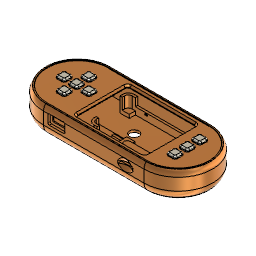
Plus_Reference (Autodesk Fusion 360 design; units mm, degrees)
Autodesk Fusion 360 part; units mm, degrees
note: some values were not read from the file. Chosen so that the rebuilt part matches the saved one: a side. Set by a fixed rule: which sketch regions a step uses.
(part 1 of 2)
sketch "Sketch1" plane through (0, 0, 0) normal (0, 0, 1) x (1, 0, 0)
  line L0 (42.95, 29.25) -> (-42.95, 29.25)
  arc A0 (-42.95, 29.25) -> (-42.95, -29.25) centre (-42.95, 0) ccw
  line L1 (-42.95, -29.25) -> (42.95, -29.25)
  arc A1 (42.95, -29.25) -> (42.95, 29.25) centre (42.95, 0) ccw
  line L2 (-42.95, 26.25) -> (42.95, 26.25)
  arc A2 (-42.95, 26.25) -> (-42.95, -26.25) centre (-42.95, 0) ccw
  line L3 (42.95, -26.25) -> (-42.95, -26.25)
  arc A3 (42.95, -26.25) -> (42.95, 26.25) centre (42.95, 0) ccw
extrude "Extrude1" add sketch "Sketch1" along normal blind 2.5 contours L2 A2 L3 A3 makes body 1
extrude "Extrude2" add sketch "Sketch1" along normal blind 22.25 bodies 1
sketch "Sketch2" plane through (0, 0, 2.5) normal (0, 0, 1) x (-1, 0, 0)
  arc A0 (42.95, -26.25) -> (42.95, 26.25) centre (42.95, 0) ccw
  line L0 (42.95, 26.25) -> (-42.95, 26.25)
  arc A1 (-42.95, 26.25) -> (-42.95, -26.25) centre (-42.95, 0) ccw
  line L1 (-42.95, -26.25) -> (42.95, -26.25)
  circle A2 centre (2.5662, -7.8588) radius 4
  arc A3 (-40.2014, 10.4179) -> (-45.3243, 5.1694) centre (-40.0743, 5.1694) ccw
  line L2 (-40.1743, 8.4179) -> (18.6467, 8.4179)
  arc A4 (-40.1743, 8.4179) -> (-43.3243, 5.1694) centre (-40.0743, 5.1694) ccw
  arc A5 (21.8967, 5.1679) -> (18.6467, 8.4179) centre (18.6467, 5.1679) ccw
  line L3 (15.8967, -22.2291) -> (15.8967, 10.4179)
  line L4 (-37.3243, -22.2291) -> (-37.3243, -24.2291)
  line L5 (-37.3243, -16.9791) -> (-37.3243, -22.2291)
  line L6 (15.8967, -22.2291) -> (15.8967, -24.2291)
  line L7 (-43.3243, -16.9791) -> (-37.3243, -16.9791)
  line L8 (21.8967, -18.9791) -> (21.8967, -15.0806)
  arc A6 (23.8967, 5.1679) -> (18.6467, 10.4179) centre (18.6467, 5.1679) ccw
  line L9 (-37.3243, -22.2291) -> (-37.3243, 10.4179)
  line L10 (-43.3243, -16.9791) -> (21.8967, -16.9791) construction
  line L11 (23.8967, -3.0806) -> (23.8967, 5.1679)
  line L12 (-40.0743, -22.2291) -> (-37.3243, -22.2291)
  line L13 (21.8967, 3.1694) -> (23.8967, 3.1694)
  line L14 (-45.3243, 3.1694) -> (-45.3243, 5.1694)
  line L15 (15.8967, -24.2291) -> (18.6467, -24.2291)
  arc A7 (18.6467, -24.2291) -> (23.8967, -18.9791) centre (18.6467, -18.9791) ccw
  line L16 (23.8967, -18.9791) -> (23.8967, -15.0806)
  line L17 (15.8967, -22.2291) -> (18.6467, -22.2291)
  line L18 (-43.3243, 3.1694) -> (21.8967, 3.1694)
  arc A8 (-45.3243, -18.9791) -> (-40.0743, -24.2291) centre (-40.0743, -18.9791) ccw
  line L19 (-45.3243, -16.9791) -> (-45.3243, -18.9791)
  line L20 (-43.3243, 3.1694) -> (-43.3243, 5.1694)
  line L21 (-40.0743, -24.2291) -> (-37.3243, -24.2291)
  line L22 (-45.3243, 3.1694) -> (-43.3243, 3.1694)
  line L23 (21.8967, -16.9791) -> (23.8967, -16.9791)
  line L24 (-40.2014, 10.4179) -> (18.6467, 10.4179)
  line L25 (15.8967, -16.9791) -> (15.8967, -22.2291)
  line L26 (15.8967, -22.2291) -> (-37.3243, -22.2291)
  line L27 (21.8967, -3.0806) -> (21.8967, -15.0806)
  arc A9 (18.6467, -22.2291) -> (21.8967, -18.9791) centre (18.6467, -18.9791) ccw
  line L28 (15.8967, -24.2291) -> (-37.3243, -24.2291)
  arc A10 (-43.3243, -18.9791) -> (-40.0743, -22.2291) centre (-40.0743, -18.9791) ccw
  line L29 (-45.3243, -16.9791) -> (-43.3243, -16.9791)
  line L30 (21.8967, -3.0806) -> (21.8967, 5.1679)
  line L31 (23.8967, -3.0806) -> (23.8967, -15.0806)
  line L32 (-43.3243, -16.9791) -> (-43.3243, -18.9791)
  line L33 (21.8967, -16.9791) -> (15.8967, -16.9791)
  arc A11 (42.95, -23.25) -> (42.95, 23.25) centre (42.95, 0) ccw
  arc A12 (42.95, -21.25) -> (42.95, 21.25) centre (42.95, 0) ccw
  arc A13 (-42.95, 23.25) -> (-42.95, -23.25) centre (-42.95, 0) ccw
  arc A14 (-42.95, 21.25) -> (-42.95, -21.25) centre (-42.95, 0) ccw
  line L34 (42.95, -23.25) -> (42.95, -21.25)
  line L35 (42.95, 21.25) -> (42.95, 23.25)
  line L36 (-42.95, 21.25) -> (-42.95, 23.25)
  line L37 (-42.95, 0) -> (-63.0851, -11.625)
  line L38 (-42.95, 0) -> (-19.7, 0) construction
  line L39 (-42.95, 0) -> (-63.0851, 11.625)
  line L40 (-42.95, 0) -> (-19.7, 0) construction
  line L41 (42.95, 0) -> (63.0851, -11.625)
  line L42 (42.95, 0) -> (66.2, 0) construction
  line L43 (42.95, 0) -> (63.0851, 11.625)
  line L44 (42.95, 0) -> (66.2, 0) construction
  line L45 (-16.3504, 12.3135) -> (-13.7656, 12.3135)
  arc A15 (-13.7656, 12.3135) -> (-13.7656, 17.551) centre (-14.2529, 14.9323) ccw
  line L46 (-13.7656, 17.551) -> (-16.0557, 17.6179)
  line L47 (-16.0557, 17.6179) -> (-16.4158, 18.1418)
  line L48 (-39.6855, 12.3135) -> (-37.1008, 12.3135)
  arc A16 (-39.6855, 17.551) -> (-39.6855, 12.3135) centre (-39.1982, 14.9323) ccw
  line L49 (-37.3955, 17.6179) -> (-39.6855, 17.551)
  line L50 (-37.0353, 18.1418) -> (-37.3955, 17.6179)
  line L51 (-16.3504, 12.3135) -> (-16.3504, 10.4179)
  line L52 (-37.1008, 12.3135) -> (-37.1008, 10.4179)
  line L53 (-16.4158, 18.1418) -> (-16.4158, 26.25)
  line L54 (-37.0353, 18.1418) -> (-37.0353, 26.25)
  line L55 (-9.4158, 26.25) -> (-9.4158, 10.4179)
  line L56 (-44.0353, 23.2247) -> (-44.0353, 26.2276)
  line L57 (-44.0353, 21.2223) -> (-44.0353, 8.6151)
  point P0 (-42.95, 0)
  point P1 (-45.1535, 0.568)
  dimension "d5" = 2
  dimension "d6" = 6
  dimension "d7" = 6
  dimension "d8" = 8
  dimension "d11" = -3
  dimension "d12" = -5
  dimension "d13" = -3
  dimension "d14" = -5
  dimension "d15" = 150
  dimension "d16" = 150
  dimension "d17" = 30
  dimension "d18" = 30
  constraint parallel L8 L27
  constraint perpendicular L20 L22
  constraint perpendicular L29 L32
  constraint coincident L13.start L30
  constraint perpendicular L18 L30
  constraint coincident L10.end L8
  constraint perpendicular L8 L10
  constraint perpendicular L7 L32
  constraint coincident L4.start L26
  constraint coincident L4.start L12
  constraint horizontal L23
  constraint coincident L23.end L16
  constraint perpendicular L16 L23
  constraint coincident L13.end L11
  constraint perpendicular L11 L13
  constraint perpendicular L6 L28
  constraint coincident L3.end L24
  constraint perpendicular L3 L24
  constraint perpendicular L4 L28
  constraint coincident L9.end L24
  constraint perpendicular L9 L24
  constraint perpendicular L1 L34
  constraint vertical L35
  constraint vertical L36
  constraint horizontal L38
  constraint coincident P0 A1.centre
  constraint coincident A13 L37.end
  constraint horizontal L40
  constraint coincident A13 L39.end
  constraint horizontal L42
  constraint coincident A0.centre A11.centre
  constraint coincident A11 L41.end
  constraint horizontal L44
  constraint coincident A11 L43.end
  constraint vertical L51
  constraint coincident L24 L51.end
  constraint perpendicular L24 L51
  constraint vertical L52
  constraint coincident L24 L52.end
  constraint vertical L53
  constraint coincident L0 L53.end
  constraint vertical L54
  constraint coincident L0 L54.end
  constraint vertical L55
  constraint coincident L24 L55.end
  constraint coincident A1 L56.end
  constraint coincident A13 L56.start
  constraint vertical L57
  constraint coincident A14 L57.start
  constraint coincident A3 L57.end
  measures "d6" distance of L10.end L25.start
  measures "d7" distance of L7.start L5.start
  measures "d8" diameter of A2
  measures "d15" angle of L37 L38
  measures "d16" angle of L39 L40
  measures "d17" angle of L41 L42
  measures "d18" angle of L43 L44
extrude "Extrude3" add sketch "Sketch2" along normal blind 3 contours L2 L3 L9 L18 | L2 A5 L3 L18 L30 | L2 A4 L9 L18 L20 | L3 L8 L17 L25 A9 L33 | L5 L7 L9 L12 A10 L32 bodies 1
extrude "Extrude4" add sketch "Sketch2" along normal blind 12.75 contours A13 A14 L36 L39 | A8 A13 A14 L37 | L4 L12 A8 L19 L21 A10 L29 L32 | L6 L8 L15 A7 L16 L17 L23 A9 | A11 A12 L34 L41 | A11 A12 L35 L43 bodies 1
extrude "Extrude5" add sketch "Sketch2" along normal blind 7.5 contours L2 L3 L9 L24 | L2 A5 L3 A6 L11 L13 L24 L30 | A3 L2 A4 L9 L14 L20 L22 L24 bodies 1
extrude "Extrude6" add sketch "Sketch2" along normal blind 6 contours L4 L6 L26 L28 bodies 1
extrude "Extrude12" add sketch "Sketch2" along normal blind 7.5 contours L0 L24 L45 A15 L46 L47 L48 A16 L49 L50 L51 L52 L53 L54 bodies 1
extrude "Extrude13" add sketch "Sketch2" along normal blind 12.75 contours L0 L24 L45 A15 L46 L47 L51 L53 L55 | L0 A1 A3 L24 A13 A14 L36 L48 A16 L49 L50 L52 L54 L56 L57 bodies 1
extrude "Extrude16" cut sketch "Sketch2" against normal up to surface (2.5 mm away) contours A2 bodies 1
sketch "Sketch3" plane through (0, -8.4179, 0) normal (0, 1, 0) x (-1, 0, 0)
  line L0 (-40.1743, 5.5) -> (18.6467, 5.5)
  line L1 (18.6467, 5.5) -> (18.6467, 10)
  line L2 (18.6467, 10) -> (-40.1743, 10)
  line L3 (-40.1743, 10) -> (-40.1743, 5.5)
  line L4 (-27.4484, 8.7376) -> (-27.4474, 8.166)
  line L5 (-27.4484, 9.136) -> (-27.4484, 8.7376)
  arc A0 (-34.511, 6.0757) -> (-34.073, 5.8861) centre (-34.0732, 6.4861) ccw
  arc A1 (-27.6097, 7.7546) -> (-27.4474, 8.166) centre (-28.0474, 8.1649) ccw
  arc A2 (-36.2473, 8.1651) -> (-36.085, 7.7547) centre (-35.6473, 8.1651) ccw
  line L6 (3.4969, 6.2998) -> (3.4969, 10.4998)
  line L7 (-25.0533, 6.7) -> (-27.0533, 6.7)
  line L8 (-31.7563, 5.887) -> (-34.073, 5.8861)
  line L9 (15.9969, 10.4998) -> (15.9969, 6.2998)
  line L10 (-27.0533, 6.7) -> (-27.0533, 7.7)
  line L11 (-34.511, 6.0757) -> (-36.085, 7.7547)
  line L12 (-36.2473, 9.136) -> (-27.4484, 9.136)
  line L13 (15.9969, 6.2998) -> (3.4969, 6.2998)
  line L14 (-0.0033, 6.7) -> (-0.0033, 7.7)
  line L15 (1.9967, 7.7) -> (1.9967, 6.7)
  line L16 (-36.2473, 8.1651) -> (-36.2473, 9.136)
  line L17 (1.9967, 6.7) -> (-0.0033, 6.7)
  line L18 (-15.0031, 5.7998) -> (-23.5031, 5.7998)
  line L19 (-27.0533, 5.5) -> (-27.0533, 6.7) construction
  line L20 (-29.6216, 5.8861) -> (-31.7563, 5.887)
  line L21 (-15.0031, 10.0008) -> (-15.0031, 5.7998)
  line L22 (-25.0533, 7.7) -> (-25.0533, 6.7)
  line L23 (-23.5031, 10.0008) -> (-15.0031, 10.0008)
  line L24 (-27.0533, 7.7) -> (-25.0533, 7.7)
  arc A3 (-29.6216, 5.8861) -> (-29.1836, 6.0757) centre (-29.6213, 6.4861) ccw
  line L25 (-0.0033, 7.7) -> (1.9967, 7.7)
  line L26 (-27.6097, 7.7546) -> (-29.1836, 6.0757)
  line L27 (-23.5031, 5.7998) -> (-23.5031, 10.0008)
  line L28 (3.4969, 10.4998) -> (15.9969, 10.4998)
  line L29 (-40.1743, 5.5) -> (-36.7473, 5.5)
  dimension "d25" = 3.427
  dimension "d26" = 1.2
  dimension "d27" = 2
  dimension "d28" = 1
  dimension "d29" = 2
  dimension "d30" = 1
  constraint vertical L19
  constraint horizontal L17
  constraint vertical L14
  constraint horizontal L25
  constraint vertical L15
  constraint horizontal L7
  constraint vertical L10
  constraint horizontal L24
  constraint vertical L22
  measures "d25" distance of L29.end L0.start
  measures "d26" distance of L19.start L7.end
  measures "d27" distance of L14.start L15.end
  measures "d28" distance of L15.start L15.end
  measures "d29" distance of L7.end L7.start
  measures "d30" distance of L7.start L22.start
extrude "Extrude7" cut sketch "Sketch3" against normal up to surface (2 mm away) contours L2 L18 L21 L23 L27 | L2 L6 L9 L13 | L2 L6 L9 L28 | L4 L5 A0 A1 A2 L8 L11 L12 L16 L20 A3 L26 bodies 1
extrude "Extrude8" add sketch "Sketch3" along normal blind 0.5 contours L7 L10 L22 L24 | L14 L15 L17 L25 bodies 1
sketch "Sketch4" plane through (0, 22.2291, 0) normal (0, -1, 0) x (1, 0, 0)
  line L0 (-18.6467, 5.5) -> (-15.8967, 5.5)
  line L1 (-15.8967, 5.5) -> (-15.8967, 2.5)
  line L2 (-15.8967, 2.5) -> (37.3243, 2.5)
  line L3 (37.3243, 2.5) -> (37.3243, 5.5)
  line L4 (37.3243, 5.5) -> (40.0743, 5.5)
  line L5 (40.0743, 5.5) -> (40.0743, 15.25)
  line L6 (40.0743, 15.25) -> (37.3243, 15.25)
  line L7 (37.3243, 15.25) -> (37.3243, 8.5)
  line L8 (37.3243, 8.5) -> (-15.8967, 8.5)
  line L9 (-15.8967, 8.5) -> (-15.8967, 15.25)
  line L10 (-15.8967, 15.25) -> (-18.6467, 15.25)
  line L11 (-18.6467, 15.25) -> (-18.6467, 5.5)
  line L12 (29.4019, 7.7) -> (27.4019, 7.7)
  line L13 (27.4019, 6.7) -> (29.4019, 6.7)
  line L14 (27.4019, 7.7) -> (27.4019, 6.7)
  line L15 (29.4019, 6.7) -> (29.4019, 7.7)
  line L16 (-5.5981, 7.7) -> (-7.5981, 7.7)
  line L17 (-7.5981, 6.7) -> (-5.5981, 6.7)
  line L18 (-5.5981, 6.7) -> (-5.5981, 7.7)
  line L19 (-7.5981, 7.7) -> (-7.5981, 6.7)
  line L20 (-15.8967, 5.5) -> (37.3243, 5.5) construction
  line L21 (-7.5981, 5.5) -> (-7.5981, 6.7) construction
  line L22 (27.4019, 5.5) -> (27.4019, 6.7) construction
  point P0 (-18.6467, 5.5)
  dimension "d35" = 2
  dimension "d36" = 1
  dimension "d37" = 2
  dimension "d38" = 1
  dimension "d195" = 1.2
  dimension "d196" = 1.2
  constraint horizontal L17
  constraint vertical L18
  constraint horizontal L16
  constraint vertical L19
  constraint horizontal L13
  constraint vertical L15
  constraint horizontal L12
  constraint vertical L14
  constraint coincident L0.end L1.start
  constraint coincident L3.end L4.start
  constraint coincident L20 L21.start
  constraint perpendicular L17 L21
  constraint coincident L20 L22.start
  constraint perpendicular L13 L22
  measures "d35" distance of L17.start L17.end
  measures "d36" distance of L17.start L16.end
  measures "d37" distance of L13.end L13.start
  measures "d38" distance of L13.start L12.end
  measures "d195" distance of L21.start L17.start
  measures "d196" distance of L22.start L13.start
extrude "Extrude9" add sketch "Sketch4" along normal blind 0.5 contours L12 L13 L14 L15 | L16 L17 L18 L19 bodies 1
chamfer "Chamfer1" distance 0.25 distance2 0.25 8 edges at (-6.5981, 21.7291, 7.7) (-6.5981, 21.7291, 6.7) (28.4019, 21.7291, 7.7) (28.4019, 21.7291, 6.7) (-0.9967, -7.9179, 7.7) (-0.9967, -7.9179, 6.7) (26.0533, -7.9179, 7.7) (26.0533, -7.9179, 6.7) measured on face at (-6.9314, 21.7291, 7.3667) measured on face at (-6.9314, 21.7291, 7.3667) measured on face at (28.0686, 21.7291, 7.3667) measured on face at (28.0686, 21.7291, 7.3667) measured on face at (-0.6634, -7.9179, 7.3667) measured on face at (-0.6634, -7.9179, 7.3667) measured on face at (25.7199, -7.9179, 7.0333) measured on face at (25.7199, -7.9179, 7.0333) on bodies 1
sketch "Sketch5" plane through (0, -29.25, 0) normal (0, -1, 0) x (1, 0, 0)
  line L0 (-42.95, 0) -> (42.95, 0)
  line L1 (42.95, 0) -> (42.95, 22.25)
  line L2 (42.95, 22.25) -> (-42.95, 22.25)
  line L3 (-42.95, 22.25) -> (-42.95, 0)
  line L4 (-37.1145, 15.75) -> (-26.7027, 15.75)
  line L5 (-37.1145, 11.75) -> (-37.1145, 15.75)
  line L6 (-26.7027, 15.75) -> (-26.7027, 11.75)
  line L7 (-37.1145, 11.75) -> (-26.7027, 11.75)
  line L8 (-37.1145, 17.95) -> (-26.7027, 17.95)
  line L9 (-37.1145, 9.55) -> (-26.7027, 9.55)
  line L10 (-24.7027, 16.95) -> (-24.7027, 10.55)
  line L11 (-39.1145, 10.55) -> (-39.1145, 16.95)
  line L12 (-39.1145, 16.95) -> (-38.1145, 16.95) construction
  line L13 (-24.7027, 16.95) -> (-25.7027, 16.95) construction
  line L14 (-24.7027, 10.55) -> (-25.7027, 10.55) construction
  line L15 (-39.1145, 10.55) -> (-38.1145, 10.55) construction
  arc A0 (-38.1145, 17.95) -> (-39.1145, 16.95) centre (-38.1145, 16.95) ccw
  line L16 (-38.1145, 16.95) -> (-38.1145, 17.95) construction
  line L17 (-38.1145, 16.95) -> (-39.1145, 16.95) construction
  arc A1 (-39.1145, 10.55) -> (-38.1145, 9.55) centre (-38.1145, 10.55) ccw
  line L18 (-38.1145, 10.55) -> (-39.1145, 10.55) construction
  line L19 (-38.1145, 10.55) -> (-38.1145, 9.55) construction
  arc A2 (-24.7027, 16.95) -> (-25.7027, 17.95) centre (-25.7027, 16.95) ccw
  line L20 (-25.7027, 16.95) -> (-24.7027, 16.95) construction
  line L21 (-25.7027, 16.95) -> (-25.7027, 17.95) construction
  arc A3 (-25.7027, 9.55) -> (-24.7027, 10.55) centre (-25.7027, 10.55) ccw
  line L22 (-25.7027, 10.55) -> (-25.7027, 9.55) construction
  line L23 (-25.7027, 10.55) -> (-24.7027, 10.55) construction
  line L24 (-25.7027, 9.55) -> (-26.7027, 9.55)
  line L25 (-38.1145, 9.55) -> (-37.1145, 9.55)
  line L26 (-38.1145, 17.95) -> (-37.1145, 17.95)
  line L27 (-25.7027, 17.95) -> (-26.7027, 17.95)
  line L28 (20.5143, 10.75) -> (33.3635, 10.75)
  line L29 (20.5143, 10.75) -> (20.5143, 13)
  line L30 (33.3635, 10.75) -> (33.3635, 13)
  line L31 (20.5143, 13) -> (33.3635, 13)
  dimension "d43" = -2.2
  dimension "d44" = 2.2
  dimension "d45" = -2
  dimension "d46" = -2
  dimension "d47" = 1
  dimension "d48" = 1
  dimension "d49" = 1
  dimension "d50" = 1
  dimension "d51" = 90
  dimension "d52" = 90
  dimension "d53" = 90
  dimension "d54" = 90
  dimension "d55" = 2.25
  dimension "d56" = 2.25
  constraint perpendicular L6 L7
  constraint perpendicular L11 L12
  constraint perpendicular L10 L13
  constraint perpendicular L10 L14
  constraint perpendicular L5 L15
  constraint coincident L12.end A0.centre
  constraint coincident L15.end A1.centre
  constraint coincident L13.end A2.centre
  constraint coincident L14.end A3.centre
  constraint tangent A3 L24
  constraint tangent A1 L25
  constraint tangent A0 L26
  constraint tangent A2 L27
  constraint vertical L29
  constraint perpendicular L28 L29
  constraint vertical L30
  measures "d47" distance of L11.end L12.end
  measures "d48" distance of L10.start L13.end
  measures "d49" distance of L10.end L14.end
  measures "d50" distance of L11.start L15.end
  measures "d51" angle of L16 L17
  measures "d52" angle of L18 L19
  measures "d53" angle of L20 L21
  measures "d54" angle of L22 L23
  measures "d55" distance of L28.start L29.end
  measures "d56" distance of L28.end L30.end
extrude "Extrude10" cut sketch "Sketch5" against normal up to surface (3 mm away) contours L4 L5 L6 L7 | L28 L29 L30 L31 bodies 1
extrude "Extrude11" cut sketch "Sketch5" against normal blind 2 contours L8 L9 L10 L11 A0 A1 A2 A3 L24 L25 L26 L27 bodies 1
fillet "Fillet4" radius 0.75 4 edges at (-37.1145, -26.75, 11.75) (-26.7027, -26.75, 11.75) (-26.7027, -26.75, 15.75) (-37.1145, -26.75, 15.75) on bodies 1
chamfer "Chamfer2" distance 3.5 distance2 3.5 4 edges at (0, -29.25, 0) (72.2, 0, 0) (0, 29.25, 0) (-72.2, 0, 0) measured on face at (-8.4536, -29.25, 3.2034) measured on face at (69.6115, 12.0301, 7.4167) measured on face at (14.3167, 29.25, 14.8333) measured on face at (-64.8811, -19.3543, 14.8333) on bodies 1
fillet "Fillet1" radius 9 4 edges at (0, 29.25, 3.5) (72.2, 0, 3.5) (0, -29.25, 3.5) (-72.2, 0, 3.5) on bodies 1
chamfer "Chamfer3" distance 2 distance2 2 4 edges at (0, -29.25, 22.25) (72.2, 0, 22.25) (0, 29.25, 22.25) (-72.2, 0, 22.25) measured on face at (12.7385, -29.25, 17.697) measured on face at (69.3147, -12.6675, 17.2426) measured on face at (14.3167, 29.25, 12.2353) measured on face at (-69.3147, 12.6675, 17.2426) on bodies 1
fillet "Fillet2" radius 6.5 4 edges at (0, -29.25, 20.25) (72.2, 0, 20.25) (0, 29.25, 20.25) (-72.2, 0, 20.25) on bodies 1
ref_plane "WorkPlane1" through (0, 0, 21.75) normal (0, 0, 1) x (1, 0, 0)
sketch "Sketch7" plane through (0, 0, 21.75) normal (0, 0, 1) x (1, 0, 0)
  line L0 (-42.95, 26.25) -> (42.95, 26.25)
  arc A0 (-42.95, 26.25) -> (-42.95, -26.25) centre (-42.95, 0) ccw
  line L1 (42.95, -26.25) -> (-42.95, -26.25)
  arc A1 (42.95, -26.25) -> (42.95, 26.25) centre (42.95, 0) ccw
  arc A2 (42.95, -26.15) -> (42.95, 26.15) centre (42.95, 0) ccw
  line L2 (-42.95, 26.15) -> (42.95, 26.15)
  arc A3 (-42.95, 26.15) -> (-42.95, -26.15) centre (-42.95, 0) ccw
  line L3 (42.95, -26.15) -> (-42.95, -26.15)
  line L4 (47.6422, 15.5801) -> (51.6422, 15.5801)
  arc A4 (47.6422, 15.5801) -> (45.6422, 13.5801) centre (47.6422, 13.5801) ccw
  line L5 (45.6422, 9.5801) -> (45.6422, 13.5801)
  arc A5 (45.6422, 9.5801) -> (47.6422, 7.5801) centre (47.6422, 9.5801) ccw
  line L6 (51.6422, 7.5801) -> (47.6422, 7.5801)
  arc A6 (51.6422, 7.5801) -> (53.6422, 9.5801) centre (51.6422, 9.5801) ccw
  line L7 (53.6422, 13.5801) -> (53.6422, 9.5801)
  arc A7 (53.6422, 13.5801) -> (51.6422, 15.5801) centre (51.6422, 13.5801) ccw
  line L8 (47.6422, 5.0801) -> (51.6422, 5.0801)
  arc A8 (47.6422, 5.0801) -> (45.6422, 3.0801) centre (47.6422, 3.0801) ccw
  line L9 (45.6422, -0.9199) -> (45.6422, 3.0801)
  arc A9 (45.6422, -0.9199) -> (47.6422, -2.9199) centre (47.6422, -0.9199) ccw
  line L10 (51.6422, -2.9199) -> (47.6422, -2.9199)
  arc A10 (51.6422, -2.9199) -> (53.6422, -0.9199) centre (51.6422, -0.9199) ccw
  line L11 (53.6422, 3.0801) -> (53.6422, -0.9199)
  arc A11 (53.6422, 3.0801) -> (51.6422, 5.0801) centre (51.6422, 3.0801) ccw
  line L12 (47.6422, -5.4199) -> (51.6422, -5.4199)
  arc A12 (47.6422, -5.4199) -> (45.6422, -7.4199) centre (47.6422, -7.4199) ccw
  line L13 (45.6422, -11.4199) -> (45.6422, -7.4199)
  arc A13 (45.6422, -11.4199) -> (47.6422, -13.4199) centre (47.6422, -11.4199) ccw
  line L14 (51.6422, -13.4199) -> (47.6422, -13.4199)
  arc A14 (51.6422, -13.4199) -> (53.6422, -11.4199) centre (51.6422, -11.4199) ccw
  line L15 (53.6422, -7.4199) -> (53.6422, -11.4199)
  arc A15 (53.6422, -7.4199) -> (51.6422, -5.4199) centre (51.6422, -7.4199) ccw
  line L16 (-46.1416, 14.6792) -> (-42.1416, 14.6792)
  arc A16 (-46.1416, 14.6792) -> (-48.1416, 12.6792) centre (-46.1416, 12.6792) ccw
  line L17 (-48.1416, 8.6792) -> (-48.1416, 12.6792)
  arc A17 (-48.1416, 8.6792) -> (-46.1416, 6.6792) centre (-46.1416, 8.6792) ccw
  line L18 (-42.1416, 6.6792) -> (-46.1416, 6.6792)
  arc A18 (-42.1416, 6.6792) -> (-40.1416, 8.6792) centre (-42.1416, 8.6792) ccw
  line L19 (-40.1416, 12.6792) -> (-40.1416, 8.6792)
  arc A19 (-40.1416, 12.6792) -> (-42.1416, 14.6792) centre (-42.1416, 12.6792) ccw
  line L20 (-46.1416, 4.1792) -> (-42.1416, 4.1792)
  arc A20 (-46.1416, 4.1792) -> (-48.1416, 2.1792) centre (-46.1416, 2.1792) ccw
  line L21 (-48.1416, -1.8208) -> (-48.1416, 2.1792)
  arc A21 (-48.1416, -1.8208) -> (-46.1416, -3.8208) centre (-46.1416, -1.8208) ccw
  line L22 (-42.1416, -3.8208) -> (-46.1416, -3.8208)
  arc A22 (-42.1416, -3.8208) -> (-40.1416, -1.8208) centre (-42.1416, -1.8208) ccw
  line L23 (-40.1416, 2.1792) -> (-40.1416, -1.8208)
  arc A23 (-40.1416, 2.1792) -> (-42.1416, 4.1792) centre (-42.1416, 2.1792) ccw
  arc A24 (-35.5416, 4.1792) -> (-37.5416, 2.1792) centre (-35.5416, 2.1792) ccw
  line L24 (-37.5416, -1.8208) -> (-37.5416, 2.1792)
  arc A25 (-37.5416, -1.8208) -> (-35.5416, -3.8208) centre (-35.5416, -1.8208) ccw
  line L25 (-31.5416, -3.8208) -> (-35.5416, -3.8208)
  arc A26 (-31.5416, -3.8208) -> (-29.5416, -1.8208) centre (-31.5416, -1.8208) ccw
  line L26 (-29.5416, 2.1792) -> (-29.5416, -1.8208)
  arc A27 (-29.5416, 2.1792) -> (-31.5416, 4.1792) centre (-31.5416, 2.1792) ccw
  line L27 (-35.5416, 4.1792) -> (-31.5416, 4.1792)
  line L28 (-46.1416, -6.3208) -> (-42.1416, -6.3208)
  arc A28 (-46.1416, -6.3208) -> (-48.1416, -8.3208) centre (-46.1416, -8.3208) ccw
  line L29 (-48.1416, -12.3208) -> (-48.1416, -8.3208)
  arc A29 (-48.1416, -12.3208) -> (-46.1416, -14.3208) centre (-46.1416, -12.3208) ccw
  line L30 (-42.1416, -14.3208) -> (-46.1416, -14.3208)
  arc A30 (-42.1416, -14.3208) -> (-40.1416, -12.3208) centre (-42.1416, -12.3208) ccw
  line L31 (-40.1416, -8.3208) -> (-40.1416, -12.3208)
  arc A31 (-40.1416, -8.3208) -> (-42.1416, -6.3208) centre (-42.1416, -8.3208) ccw
  line L32 (-50.7416, 2.1792) -> (-50.7416, -1.8208)
  arc A32 (-50.7416, 2.1792) -> (-52.7416, 4.1792) centre (-52.7416, 2.1792) ccw
  line L33 (-56.7416, 4.1792) -> (-52.7416, 4.1792)
  arc A33 (-56.7416, 4.1792) -> (-58.7416, 2.1792) centre (-56.7416, 2.1792) ccw
  line L34 (-58.7416, -1.8208) -> (-58.7416, 2.1792)
  arc A34 (-58.7416, -1.8208) -> (-56.7416, -3.8208) centre (-56.7416, -1.8208) ccw
  line L35 (-52.7416, -3.8208) -> (-56.7416, -3.8208)
  arc A35 (-52.7416, -3.8208) -> (-50.7416, -1.8208) centre (-52.7416, -1.8208) ccw
  line L36 (-22.4574, -20.4312) -> (-22.4574, 20.174)
  arc A36 (-20.4574, 22.174) -> (-22.4574, 20.174) centre (-20.4574, 20.174) ccw
  line L37 (-20.4574, 22.174) -> (34.5431, 22.174)
  line L38 (36.5431, 20.174) -> (36.5431, -20.4312)
  arc A37 (36.5431, 20.174) -> (34.5431, 22.174) centre (34.5431, 20.174) ccw
  arc A38 (34.5431, -22.4312) -> (36.5431, -20.4312) centre (34.5431, -20.4312) ccw
  line L39 (34.5431, -22.4312) -> (-20.4574, -22.4312)
  arc A39 (-22.4574, -20.4312) -> (-20.4574, -22.4312) centre (-20.4574, -20.4312) ccw
  arc A40 (-42.95, 23.25) -> (-42.95, -23.25) centre (-42.95, 0) ccw
  arc A41 (42.95, -23.25) -> (42.95, 23.25) centre (42.95, 0) ccw
  arc A42 (42.95, -21.25) -> (42.95, 21.25) centre (42.95, 0) ccw
  arc A43 (-42.95, 21.25) -> (-42.95, -21.25) centre (-42.95, 0) ccw
  line L40 (-54.575, 20.1351) -> (-53.575, 18.403)
  line L41 (-63.0851, 11.625) -> (-61.353, 10.625)
  line L42 (-63.0851, -11.625) -> (-61.353, -10.625)
  line L43 (-54.575, -20.1351) -> (-53.575, -18.403)
  line L44 (56.6092, 16.2784) -> (57.9609, 17.8893)
  line L45 (57.9609, 17.8893) -> (56.6092, 16.2784)
  line L46 (64.7979, 7.952) -> (62.9185, 7.2679)
  line L47 (64.7979, -7.952) -> (62.9185, -7.2679)
  line L48 (56.6092, -16.2784) -> (57.8948, -17.8105)
  arc A44 (-42.95, 25.65) -> (-42.95, -25.65) centre (-42.95, 0) ccw
  line L49 (-42.95, -25.65) -> (-42.95, -26.25)
  line L50 (-45.0332, -25.5653) -> (-45.0925, -26.1624)
  line L51 (45.6422, 13.5801) -> (45.6422, 23.0936)
  line L52 (45.6422, -11.4199) -> (45.6422, -23.0936)
  arc A45 (-63.0851, -11.625) -> (-54.575, -20.1351) centre (-42.95, 0) ccw
  arc A46 (-61.353, -10.625) -> (-53.575, -18.403) centre (-42.95, 0) ccw
  line L53 (-42.95, -23.25) -> (-29.5416, -23.25)
  line L54 (-29.5416, -23.25) -> (-29.5416, -9.3208)
  line L55 (-29.5416, -9.3208) -> (-31.5416, -9.3208)
  line L56 (-31.5416, -9.3208) -> (-31.5416, -21.2498)
  line L57 (-31.5416, -21.2498) -> (-42.95, -21.25)
  line L58 (-42.95, -21.25) -> (-42.95, -23.25)
  line L59 (-42.95, 23.25) -> (-29.5416, 23.25)
  line L60 (-29.5416, 23.25) -> (-29.5416, 9.321)
  line L61 (-29.5416, 9.321) -> (-31.5416, 9.321)
  line L62 (-31.5416, 9.321) -> (-31.5416, 21.25)
  line L63 (-31.5416, 21.25) -> (-42.95, 21.25)
  line L64 (-42.95, 21.25) -> (-42.95, 23.25)
  line L65 (-24.3116, 24.4286) -> (43.6884, 24.4286)
  line L66 (-24.3116, -23.7714) -> (-24.3116, 24.4286)
  line L67 (43.6884, -23.7714) -> (-24.3116, -23.7714)
  line L68 (0, 0) -> (-24.3116, 0) construction
  line L69 (43.6884, 24.4286) -> (43.6884, -23.7714)
  line L70 (44.6884, -24.7714) -> (-25.3116, -24.7714)
  line L71 (-25.3116, -24.7714) -> (-25.3116, 25.4286)
  line L72 (-25.3116, 25.4286) -> (44.6884, 25.4286)
  line L73 (44.6884, 25.4286) -> (44.6884, -24.7714)
  line L74 (44.6884, 25.4286) -> (39.6884, 25.4286) construction
  line L75 (44.6884, 25.4286) -> (44.6884, 20.4286) construction
  line L76 (44.6884, -24.7714) -> (44.6884, -19.7714) construction
  line L77 (44.6884, -24.7714) -> (39.6884, -24.7714) construction
  line L78 (-25.3116, -24.7714) -> (-20.3116, -24.7714) construction
  line L79 (-25.3116, -24.7714) -> (-25.3116, -19.7714) construction
  line L80 (-25.3116, 25.4286) -> (-20.3116, 25.4286) construction
  line L81 (-25.3116, 25.4286) -> (-25.3116, 20.4286) construction
  line L82 (-20.3116, 25.4286) -> (-20.3116, 24.4286)
  line L83 (-25.3116, 20.4286) -> (-24.3116, 20.4286)
  line L84 (-25.3116, -19.7714) -> (-24.3116, -19.7714)
  line L85 (-20.3116, -24.7714) -> (-20.3116, -23.7714)
  line L86 (39.6884, -24.7714) -> (39.6884, -23.7714)
  line L87 (44.6884, -19.7714) -> (43.6884, -19.7714)
  line L88 (39.6884, 25.4286) -> (39.6884, 24.4286)
  line L89 (44.6884, 20.4286) -> (43.6884, 20.4286)
  point P0 (-42.95, 26.25)
  point P1 (-42.95, 26.25)
  dimension "d79" = 0.1
  dimension "d168" = -0.6
  dimension "d173" = 2
  dimension "d176" = 2
  dimension "d197" = -1
  dimension "d198" = 5
  dimension "d199" = 5
  dimension "d200" = 5
  dimension "d201" = 5
  dimension "d202" = 5
  dimension "d203" = 5
  dimension "d204" = 5
  dimension "d205" = 5
  constraint coincident L40.start A40
  constraint coincident L41.start A40
  constraint coincident L43.start A40
  constraint coincident L42.start A40
  constraint coincident L46.start A41
  constraint coincident L47.start A41
  constraint coincident A43 L40.end
  constraint coincident A43 L41.end
  constraint coincident A43 L42.end
  constraint coincident A43 L43.end
  constraint coincident A42 L44.start
  constraint coincident A42 L46.end
  constraint coincident A42 L47.end
  constraint coincident A42 L48.start
  constraint coincident A41 L48.end
  constraint coincident A0.end L1.end
  constraint perpendicular L1 L49
  constraint coincident A44 L50.start
  constraint coincident A0 L50.end
  constraint vertical L51
  constraint coincident A41 L51.end
  constraint tangent A4 L51
  constraint vertical L52
  constraint coincident A41 L52.end
  constraint tangent A13 L52
  constraint coincident A0.centre A3.centre
  constraint tangent A40 L53
  constraint perpendicular L26 L53
  constraint perpendicular L28 L54
  constraint perpendicular L54 L55
  constraint perpendicular L55 L56
  constraint perpendicular L53 L58
  constraint tangent A40 L59
  constraint perpendicular L26 L59
  constraint perpendicular L59 L60
  constraint perpendicular L60 L61
  constraint perpendicular L61 L62
  constraint tangent A43 L63
  constraint perpendicular L59 L64
  constraint coincident L68.end L66
  constraint perpendicular L67 L69
  constraint perpendicular L73 L74
  constraint perpendicular L72 L75
  constraint perpendicular L70 L76
  constraint perpendicular L73 L77
  constraint perpendicular L71 L78
  constraint perpendicular L78 L79
  constraint perpendicular L71 L80
  constraint perpendicular L80 L81
  constraint coincident L65 L82.end
  constraint perpendicular L65 L82
  constraint coincident L66 L83.end
  constraint perpendicular L66 L83
  constraint coincident L66 L84.end
  constraint perpendicular L66 L84
  constraint coincident L67 L85.end
  constraint perpendicular L67 L85
  constraint coincident L67 L86.end
  constraint perpendicular L67 L86
  constraint coincident L69 L87.end
  constraint perpendicular L69 L87
  constraint coincident L65 L88.end
  constraint perpendicular L65 L88
  constraint coincident L69 L89.end
  constraint perpendicular L69 L89
  measures "d173" distance of L54.end L55.end
  measures "d176" distance of L60.end L61.end
  measures "d198" distance of L72.end L74.end
  measures "d199" distance of L72.end L75.end
  measures "d200" distance of L70.start L76.end
  measures "d201" distance of L70.start L77.end
  measures "d202" distance of L70.end L78.end
  measures "d203" distance of L70.end L79.end
  measures "d204" distance of L71.end L80.end
  measures "d205" distance of L71.end L81.end
extrude "Extrude15" add sketch "Sketch7" against normal blind 2 separate body contours A2 L2 A3 L3 A44 L49 L50 | A40 A43 L40 L64 | L59 L60 L61 L62 L63 L64 | A40 A43 L41 L42 | A40 A43 L43 L58 | L53 L54 L55 L56 L57 L58 | A41 A42 L48 L52 | A41 A42 L52 L73 | A42 L73 | A41 A42 L46 L47 | L65 L66 L67 L69 | L69 L73 L87 L89 | L67 L70 L85 L86 | A41 A42 L44 L45 L51 | A41 A42 L51 L73 | L66 L71 L83 L84 | L65 L72 L82 L88 makes body 2
extrude "Extrude17" add sketch "Sketch7" against normal blind 4.8 contours L59 L60 L61 L62 L63 L64 | A40 A43 L40 L41 | A40 A43 L41 L42 | A40 A43 L42 L43 A45 A46 | L53 L54 L55 L56 L57 L58 | A41 A42 L48 L52 | A41 A42 L47 L48 | A41 A42 L44 L45 L46 | A41 A42 L44 L45 L51 bodies 2
extrude "Extrude26" add sketch "Sketch7" against normal blind 3.4 contours A41 L67 L69 L70 L73 L86 | A41 A42 L69 L73 | A42 L69 L73 L87 | A42 L69 L73 L89 | L66 L67 L70 L71 L84 L85 | A41 A42 L69 L73 | A41 L65 L69 L72 L73 L88 | L65 L66 L71 L72 L82 L83 bodies 2
chamfer "Chamfer4" distance 1.4 distance2 1.4 8 edges at (7.0429, 22.174, 21.75) (35.9573, 21.5882, 21.75) (36.5431, -0.1286, 21.75) (35.9573, -21.8454, 21.75) (7.0429, -22.4312, 21.75) (-21.8716, -21.8454, 21.75) (-22.4574, -0.1286, 21.75) (-21.8716, 21.5882, 21.75) measured on face at (-31.2921, -12.279, 21.75) measured on face at (-31.2921, -12.279, 21.75) measured on face at (-31.2921, -12.279, 21.75) measured on face at (-31.2921, -12.279, 21.75) measured on face at (-31.2921, -12.279, 21.75) measured on face at (-31.2921, -12.279, 21.75) measured on face at (-31.2921, -12.279, 21.75) measured on face at (-31.2921, -12.279, 21.75) on bodies 2
sketch "Sketch8" plane through (0, 0, 13) normal (0, 0, -1) x (1, 0, 0)
  line L0 (20.5143, 26.25) -> (33.3635, 26.25)
  line L1 (33.3635, 26.25) -> (33.3635, 29.25)
  line L2 (33.3635, 29.25) -> (20.5143, 29.25)
  line L3 (20.5143, 29.25) -> (20.5143, 26.25)
  line L4 (33.3635, 26.25) -> (20.5143, 26.25) construction
  line L5 (26.9389, 26.25) -> (26.9389, 26.75) construction
  arc A0 (20.5143, 29.25) -> (33.3635, 29.25) centre (26.9389, 36.2551) ccw
  dimension "d92" = 0.5
  constraint vertical L5
  constraint midpoint L0 L5.start
  constraint coincident L5.end A0
  constraint coincident L1.end L2.start
  constraint coincident L2.end L3.start
  measures "d92" distance of L5.start L5.end
sketch "Sketch10" plane through (0, 0, 10.75) normal (0, 0, 1) x (-1, 0, 0)
  line L0 (-33.3635, 26.25) -> (-20.5143, 26.25)
  line L1 (-20.5143, 26.25) -> (-20.5143, 29.25)
  line L2 (-20.5143, 29.25) -> (-33.3635, 29.25)
  line L3 (-33.3635, 29.25) -> (-33.3635, 26.25)
  line L4 (-20.5143, 26.25) -> (-33.3635, 26.25)
  line L5 (-33.3635, 29.25) -> (-20.5143, 29.25)
  line L6 (-26.9389, 26.25) -> (-26.9389, 26.75) construction
  arc A0 (-33.3635, 29.25) -> (-20.5143, 29.25) centre (-26.9389, 36.2551) ccw
  dimension "d101" = 0.5
  constraint vertical L6
  constraint midpoint L4 L6.start
  constraint coincident L6.end A0
  constraint coincident L2.end L3.start
  constraint coincident L1.end L2.start
  measures "d101" distance of L6.start L6.end
ref_plane "WorkPlane2" through (26.9389, -27.75, 11.875) normal (-1, 0, 0) x (0, 0, 1)
sketch "Sketch9" plane through (26.9389, 0, 0) normal (-1, 0, 0) x (0, -1, 0)
  line L0 (29.25, 13) -> (34.25, 21.6603)
  line L1 (29.25, 13) -> (39.25, 13) construction
  line L2 (29.25, 10.75) -> (35.4066, 2.8699)
  line L3 (29.25, 10.75) -> (39.25, 10.75) construction
  point P0 (29.25, 13)
  point P1 (29.25, 10.75)
  dimension "d93" = 10
  dimension "d94" = 60
  dimension "d102" = 10
  dimension "d103" = 52
  constraint horizontal L1
  constraint coincident P0 L0.start
  constraint horizontal L3
  constraint coincident P1 L2.start
  measures "d93" distance of P0 L0.end
  measures "d94" angle of L0 L1
  measures "d102" distance of P1 L2.end
  measures "d103" angle of L2 L3
sweep "Sweep1" cut profiles "Sketch8" path "Sketch9" along L0 section 1 contours L2 A0 bodies 1
sweep "Sweep2" cut profiles "Sketch10" path "Sketch9" along L2 section 1 contours L2 L5 A0 bodies 1
ref_plane "WorkPlane3" through (42.95, 26.15, 20.75) normal (1, 0, 0) x (0, 0, -1)
sketch "Sketch11" plane through (42.95, 0, 0) normal (1, 0, 0) x (0, 1, 0)
  line L0 (26.15, 21.75) -> (26.15, 19.75)
  line L1 (26.15, 21.75) -> (26.15, 19.75)
  line L2 (26.15, 20.75) -> (26.15, 21.5)
  line L3 (26.15, 20.75) -> (26.15, 20)
  line L4 (26.15, 21.5) -> (29.15, 21.5) construction
  line L5 (26.15, 20) -> (26.9, 20.75)
  line L6 (26.15, 20) -> (27.2107, 20) construction
  line L7 (26.15, 21.5) -> (26.9, 20.75)
  line L8 (-26.15, 21.75) -> (-26.15, 19.75)
  line L9 (-26.15, 20.75) -> (-26.15, 21.5)
  line L10 (-26.15, 20.75) -> (-26.15, 20)
  line L11 (-26.15, 21.5) -> (-21.15, 21.5) construction
  line L12 (-26.15, 20) -> (-26.9, 20.75)
  line L13 (-26.15, 20) -> (-25.0893, 20) construction
  line L14 (-26.15, 21.5) -> (-26.9, 20.75)
  dimension "d111" = 0.75
  dimension "d112" = 0.75
  dimension "d115" = 45
  dimension "d116" = 0.75
  dimension "d117" = 0.75
  dimension "d120" = 135
  constraint midpoint L0 L2.start
  constraint parallel L1 L2
  constraint parallel L0 L3
  constraint horizontal L4
  constraint horizontal L6
  constraint perpendicular L5 L7
  constraint midpoint L8 L9.start
  constraint parallel L8 L9
  constraint parallel L8 L10
  constraint horizontal L11
  constraint horizontal L13
  constraint perpendicular L12 L14
  measures "d111" distance of L2.start L2.end
  measures "d112" distance of L2.start L3.end
  measures "d115" angle of L5 L6
  measures "d116" distance of L9.start L9.end
  measures "d117" distance of L9.start L10.end
  measures "d120" angle of L12 L13
extrude "Extrude18" add sketch "Sketch11" against normal up to surface (85.9 mm away) bodies 2
ref_plane "WorkPlane4" through (-42.95, -26.25, 12.375) normal (-1, 0, 0) x (0, 0, 1)
sketch "Sketch12" plane through (-42.95, 0, 0) normal (-1, 0, 0) x (0, -1, 0)
  line L0 (-27.25, 22.25) -> (27.25, 22.25)
  line L1 (26.25, 22.25) -> (26.25, 21.5) construction
  line L2 (26.25, 21.5) -> (26.25, 20)
  line L3 (26.25, 21.5) -> (31.25, 21.5) construction
  line L4 (26.25, 20) -> (27, 20.75)
  line L5 (26.25, 20) -> (27.3107, 20) construction
  line L6 (26.25, 21.5) -> (27, 20.75)
  line L7 (-26.25, 22.25) -> (-26.25, 21.5) construction
  line L8 (-26.25, 21.5) -> (-26.25, 20)
  line L9 (-26.25, 21.5) -> (-23.25, 21.5) construction
  line L10 (-26.25, 20) -> (-27, 20.75)
  line L11 (-26.25, 20) -> (-25.1893, 20) construction
  line L12 (-26.25, 21.5) -> (-27, 20.75)
  point P0 (26.25, 22.25)
  point P1 (-26.25, 22.25)
  dimension "d124" = 0.75
  dimension "d125" = 1.5
  dimension "d128" = 45
  dimension "d129" = 0.75
  dimension "d130" = 1.5
  dimension "d133" = 135
  constraint coincident P0 L1.start
  constraint perpendicular L0 L1
  constraint perpendicular L0 L2
  constraint horizontal L3
  constraint horizontal L5
  constraint perpendicular L4 L6
  constraint coincident P1 L7.start
  constraint perpendicular L0 L7
  constraint perpendicular L0 L8
  constraint horizontal L9
  constraint horizontal L11
  constraint perpendicular L10 L12
  measures "d124" distance of P0 L1.end
  measures "d125" distance of L1.end L2.end
  measures "d128" angle of L4 L5
  measures "d129" distance of P1 L7.end
  measures "d130" distance of L7.end L8.end
  measures "d133" angle of L10 L11
extrude "Extrude19" cut sketch "Sketch12" against normal up to surface (85.9 mm away) bodies 1
ref_plane "WorkPlane5" through (-0.5014, 0, 19.74) normal (0, 0, -1) x (-1, 0, 0)